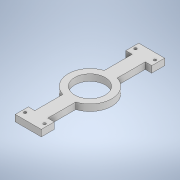
# Autodesk Inventor part: upper_grip
Saved by Autodesk Inventor 2021 (Build 250183000, 183)
## iProperties
Created: 2020-10-08
Part Number: upper_grip
Material: Generic
Document SubType Name: Modeling
Designer: bober
Density: 1 g/cm^3
Appearance: Default
Author: bober
Autodesk Inventor part; units mm, degrees
ref_plane "YZ Plane" through (0, 0, 0) normal (1, 0, 0) x (0, 1, 0)
ref_plane "XZ Plane" through (0, 0, 0) normal (0, 1, 0) x (-1, 0, 0)
ref_plane "XY Plane" through (0, 0, 0) normal (0, 0, 1) x (1, 0, 0)
sketch "Sketch1" plane through (0, 0, 0) normal (0, 1, 0) x (-1, 0, 0)
  line L0 (-10, 95) -> (10, 95)
  line L1 (10, 95) -> (10, -95)
  line L2 (10, -95) -> (-10, -95)
  line L3 (-10, -95) -> (-10, 95)
  line L4 (-10, 95) -> (10, -95) construction
  line L5 (10, 95) -> (-10, -95) construction
  line L6 (20, -95) -> (-20, -95)
  line L7 (-20, -95) -> (-20, -75)
  line L8 (-20, -75) -> (20, -75)
  line L9 (20, -75) -> (20, -95)
  line L10 (-20, 95) -> (20, 95)
  line L11 (20, 95) -> (20, 75)
  line L12 (20, 75) -> (-20, 75)
  line L13 (-20, 75) -> (-20, 95)
  point P0 (0, 0)
  point P1 (-10, 75)
  point P2 (-10, -75)
  point P3 (10, -75)
  point P4 (10, 75)
  dimension "d0" = 20
  dimension "d1" = 190
  dimension "d2" = 40
  dimension "d3" = 20
  dimension "d4" = 40
  dimension "d5" = 20
  constraints: 28 end point, 6 parallel, 3 horizontal, 3 perpendicular, 2 midpoint, 1 point on line
  measures "d0" distance of L1.end L2.end
  measures "d1" distance of L0.end L1.end
  measures "d2" distance of L7.end L8.end
  measures "d3" distance of L6.end L7.end
  measures "d4" distance of L11.end L12.end
  measures "d5" distance of L10.end L11.end
extrude "Extrusion1" add sketch "Sketch1" along normal blind 10
sketch "Sketch2" plane through (0, 10, 0) normal (0, 1, 0) x (1, 0, 0)
  circle A0 centre (0, 0) radius 23.5
  circle A1 centre (0, 0) radius 33.5
  dimension "d8" = 47
  dimension "d9" = 67
  constraints: 2 centre point, 2 coincident
  measures "d8" diameter of A0
  measures "d9" diameter of A1
extrude "Extrusion2" add sketch "Sketch2" against normal blind 10
sketch "Sketch3" plane through (0, 10, 0) normal (0, 1, 0) x (1, 0, 0)
  circle A0 centre (0, 0) radius 23.5
  constraints: 1 centre point, 1 coincident
extrude "Extrusion3" cut sketch "Sketch3" against normal blind 10
sketch "Sketch4" plane through (0, 10, 0) normal (0, 1, 0) x (1, 0, 0)
  circle A0 centre (-15, -85) radius 2
  circle A1 centre (15, -85) radius 2
  circle A2 centre (-15, 85) radius 2
  circle A3 centre (15, 85) radius 2
  point P0 (0, 0)
  dimension "d14" = 4
  dimension "d15" = 4
  dimension "d16" = 4
  dimension "d17" = 4
  constraints: 4 centre point
  measures "d14" diameter of A0
  measures "d15" diameter of A1
  measures "d16" diameter of A2
  measures "d17" diameter of A3
extrude "Extrusion4" cut sketch "Sketch4" against normal blind 10
body "Solid1"
